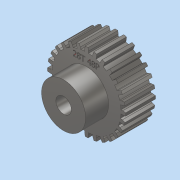
# Autodesk Inventor part: largeIdlerPinion
Saved by Autodesk Inventor 2017 (Build 210142000, 142)
## iProperties
Created: 2016-11-30
Part Number: largeIdlerPinion
Material: Steel, Carbon
Document SubType Name: Modeling
Designer: techn
Density: 7.85 g/cm^3
Appearance: Semi-Polished
Author: techn
Comments: A pinion gear i already own of the 20 to 24 tooth variety - adjust mesh in ballast section based on the axle pitch
Autodesk Inventor part; units mm, degrees
note: some values were not read from the file. Chosen so that the rebuilt part matches the saved one: direction of "Emboss1".
ref_plane "YZ Plane" through (0, 0, 0) normal (1, 0, 0) x (0, 1, 0)
ref_plane "XZ Plane" through (0, 0, 0) normal (0, 1, 0) x (-1, 0, 0)
ref_plane "XY Plane" through (0, 0, 0) normal (0, 0, 1) x (1, 0, 0)
sketch "Sketch1" plane through (0, 0, 0) normal (0, 0, 1) x (1, 0, 0)
  circle A0 centre (0, 0) radius 7.0358
  dimension "d0" = 14.0716
  constraints: 1 centre point, 1 coincident
  measures "d0" diameter of A0
extrude "Extrusion1" add sketch "Sketch1" along normal blind 6.096
sketch "Sketch2" plane through (0, 0, 6.096) normal (0, 0, 1) x (1, 0, 0)
  circle A0 centre (0, 0) radius 4.5085
  dimension "d3" = 9.017
  constraints: 1 centre point, 1 coincident
  measures "d3" diameter of A0
extrude "Extrusion2" add sketch "Sketch2" along normal blind 4.699
sketch "Sketch3" plane through (0, 0, 10.795) normal (0, 0, 1) x (1, 0, 0)
  circle A0 centre (0, 0) radius 1.5875
  dimension "d6" = 3.175
  constraints: 1 centre point, 1 coincident
  measures "d6" diameter of A0
extrude "Extrusion3" cut sketch "Sketch3" against normal blind 25.4
sketch "Sketch5" plane through (0, 0, 0) normal (0, 0, -1) x (-1, 0, 0)
  line L0 (-0.3683, 7.0262) -> (0.3683, 7.0262)
  line L1 (0.3683, 7.0262) -> (0.3683, 7.4072)
  line L2 (0.3683, 7.4072) -> (0.2921, 7.9914)
  line L3 (0.2921, 7.9914) -> (-0.2921, 7.9914)
  line L4 (-0.2921, 7.9914) -> (-0.3683, 7.4072)
  line L5 (-0.3683, 7.4072) -> (-0.3683, 7.0262)
  circle A0 centre (0, 0) radius 7.0358 projected
  point P0 (0, 7.9914)
  point P1 (0, 7.0262)
  dimension "d20" = 0.5842
  dimension "d21" = 0.7366
  dimension "d22" = 0.381
  dimension "d23" = 0.5842
  constraints: 12 end point, 2 midpoint, 2 parallel, 2 vertical alignment, 1 horizontal, 1 horizontal alignment, 1 perpendicular, 2 other
  measures "d20" distance of L2.end L3.end
  measures "d21" distance of L0.start L0.end
  measures "d22" distance of L0.end L1.end
  measures "d23" distance from line of L4.end L3
extrude "Extrusion5" add sketch "Sketch5" against normal up to surface (6.096 mm away) contours A0 L0 | L5 L4 L3 L2 L1 A0 picked at (-0.0409, 7.029)
pattern_circular "Circular Pattern1" count 28 over 360 about axis through (0, 0, 0) along (0, 0, 1) of "Extrusion5"
sketch "Sketch6" plane through (0, 0, 6.096) normal (0, 0, 1) x (1, 0, 0)
  line L0 (-2.8231, 6.1378) -> (2.6097, 6.1378) construction
  line L1 (2.6097, 6.1378) -> (2.6097, 5.0003) construction
  line L2 (2.6097, 5.0003) -> (-2.8231, 5.0003) construction
  line L3 (-2.8231, 5.0003) -> (-2.8231, 6.1378) construction
  line L4 (-2.0727, 5.025) -> (-2.7437, 5.025)
  line L5 (-2.7437, 5.025) -> (-2.7437, 5.1793)
  spline S0 degree 2 poles (-2.7437, 5.1793) (-2.6714, 5.2472) (-2.5427, 5.3733) (-2.4809, 5.4412) knots 0 0 0 1 2 2 2
  spline S1 degree 2 poles (-2.4809, 5.4412) (-2.3566, 5.5779) (-2.2658, 5.7419) (-2.2658, 5.8292) knots 0 0 0 1 2 2 2
  spline S2 degree 2 poles (-2.2658, 5.8292) (-2.2658, 5.875) (-2.294, 5.9438) (-2.3196, 5.9659) knots 0 0 0 1 2 2 2
  spline S3 degree 2 poles (-2.3196, 5.9659) (-2.3451, 5.9879) (-2.4122, 6.01) (-2.4527, 6.01) knots 0 0 0 1 2 2 2
  spline S4 degree 2 poles (-2.4527, 6.01) (-2.4915, 6.01) (-2.5709, 5.9906) (-2.607, 5.9756) knots 0 0 0 1 2 2 2
  spline S5 degree 2 poles (-2.607, 5.9756) (-2.6379, 5.9632) (-2.6952, 5.9279) (-2.7128, 5.9156) knots 0 0 0 1 2 2 2
  line L6 (-2.7128, 5.9156) -> (-2.7208, 5.9156)
  line L7 (-2.7208, 5.9156) -> (-2.7208, 6.0708)
  spline S6 degree 2 poles (-2.7208, 6.0708) (-2.6758, 6.0928) (-2.5144, 6.136) (-2.4421, 6.136) knots 0 0 0 1 2 2 2
  spline S7 degree 2 poles (-2.4421, 6.136) (-2.2896, 6.136) (-2.1176, 5.9747) (-2.1176, 5.8371) knots 0 0 0 1 2 2 2
  spline S8 degree 2 poles (-2.1176, 5.8371) (-2.1176, 5.7727) (-2.1476, 5.6652) (-2.1741, 5.6193) knots 0 0 0 1 2 2 2
  spline S9 degree 2 poles (-2.1741, 5.6193) (-2.2005, 5.5717) (-2.2772, 5.4782) (-2.3196, 5.4333) knots 0 0 0 1 2 2 2
  spline S10 degree 2 poles (-2.3196, 5.4333) (-2.3883, 5.3583) (-2.5568, 5.1978) (-2.607, 5.1511) knots 0 0 0 1 2 2 2
  line L8 (-2.607, 5.1511) -> (-2.0727, 5.1511)
  line L9 (-2.0727, 5.1511) -> (-2.0727, 5.025)
  spline S11 degree 2 poles (-1.5983, 5.0003) (-1.6794, 5.0003) (-1.8125, 5.0488) (-1.8593, 5.0938) knots 0 0 0 1 2 2 2
  spline S12 degree 2 poles (-1.8593, 5.0938) (-1.9051, 5.1379) (-1.9527, 5.2578) (-1.9527, 5.3257) knots 0 0 0 1 2 2 2
  spline S13 degree 2 poles (-1.9527, 5.3257) (-1.9527, 5.4139) (-1.8584, 5.562) (-1.7684, 5.6061) knots 0 0 0 1 2 2 2
  line L10 (-1.7684, 5.6061) -> (-1.7684, 5.6105)
  spline S14 degree 2 poles (-1.7684, 5.6105) (-1.8487, 5.6572) (-1.9263, 5.7683) (-1.9263, 5.8512) knots 0 0 0 1 2 2 2
  spline S15 degree 2 poles (-1.9263, 5.8512) (-1.9263, 5.9738) (-1.7411, 6.1378) (-1.5983, 6.1378) knots 0 0 0 1 2 2 2
  spline S16 degree 2 poles (-1.5983, 6.1378) (-1.4501, 6.1378) (-1.2711, 5.9826) (-1.2711, 5.8609) knots 0 0 0 1 2 2 2
  spline S17 degree 2 poles (-1.2711, 5.8609) (-1.2711, 5.7877) (-1.3566, 5.6449) (-1.4369, 5.6043) knots 0 0 0 1 2 2 2
  line L11 (-1.4369, 5.6043) -> (-1.4369, 5.5999)
  spline S18 degree 2 poles (-1.4369, 5.5999) (-1.3417, 5.5558) (-1.2438, 5.4288) (-1.2438, 5.3283) knots 0 0 0 1 2 2 2
  spline S19 degree 2 poles (-1.2438, 5.3283) (-1.2438, 5.189) (-1.4466, 5.0003) (-1.5983, 5.0003) knots 0 0 0 1 2 2 2
  spline S20 degree 2 poles (-1.3937, 5.3142) (-1.3937, 5.3812) (-1.4466, 5.4606) (-1.5215, 5.5012) knots 0 0 0 1 2 2 2
  spline S21 degree 2 poles (-1.5215, 5.5012) (-1.5462, 5.5153) (-1.6291, 5.5479) (-1.6811, 5.5691) knots 0 0 0 1 2 2 2
  spline S22 degree 2 poles (-1.6811, 5.5691) (-1.7411, 5.5294) (-1.8055, 5.4112) (-1.8055, 5.3363) knots 0 0 0 1 2 2 2
  spline S23 degree 2 poles (-1.8055, 5.3363) (-1.8055, 5.2375) (-1.6864, 5.1088) (-1.5965, 5.1088) knots 0 0 0 1 2 2 2
  spline S24 degree 2 poles (-1.5965, 5.1088) (-1.5048, 5.1088) (-1.3937, 5.219) (-1.3937, 5.3142) knots 0 0 0 1 2 2 2
  spline S25 degree 2 poles (-1.414, 5.8592) (-1.414, 5.9324) (-1.5118, 6.0302) (-1.5991, 6.0302) knots 0 0 0 1 2 2 2
  spline S26 degree 2 poles (-1.5991, 6.0302) (-1.6785, 6.0302) (-1.7799, 5.9429) (-1.7799, 5.868) knots 0 0 0 1 2 2 2
  spline S27 degree 2 poles (-1.7799, 5.868) (-1.7799, 5.8142) (-1.7279, 5.7392) (-1.6759, 5.7093) knots 0 0 0 1 2 2 2
  spline S28 degree 2 poles (-1.6759, 5.7093) (-1.6538, 5.6969) (-1.5603, 5.6537) (-1.5224, 5.6414) knots 0 0 0 1 2 2 2
  spline S29 degree 2 poles (-1.5224, 5.6414) (-1.4589, 5.6899) (-1.414, 5.793) (-1.414, 5.8592) knots 0 0 0 1 2 2 2
  line L12 (-0.8258, 5.025) -> (-0.8258, 5.9844)
  line L13 (-0.8258, 5.9844) -> (-1.1909, 5.9844)
  line L14 (-1.1909, 5.9844) -> (-1.1909, 6.1131)
  line L15 (-1.1909, 6.1131) -> (-0.3161, 6.1131)
  line L16 (-0.3161, 6.1131) -> (-0.3161, 5.9844)
  line L17 (-0.3161, 5.9844) -> (-0.6812, 5.9844)
  line L18 (-0.6812, 5.9844) -> (-0.6812, 5.025)
  line L19 (-0.6812, 5.025) -> (-0.8258, 5.025)
  line L20 (0.9307, 5.3989) -> (0.8011, 5.3989)
  line L21 (0.8011, 5.3989) -> (0.8011, 5.025)
  line L22 (0.8011, 5.025) -> (0.6609, 5.025)
  line L23 (0.6609, 5.025) -> (0.6609, 5.3989)
  line L24 (0.6609, 5.3989) -> (0.1803, 5.3989)
  line L25 (0.1803, 5.3989) -> (0.1803, 5.5523)
  line L26 (0.1803, 5.5523) -> (0.6671, 6.1131)
  line L27 (0.6671, 6.1131) -> (0.8011, 6.1131)
  line L28 (0.8011, 6.1131) -> (0.8011, 5.5161)
  line L29 (0.8011, 5.5161) -> (0.9307, 5.5161)
  line L30 (0.9307, 5.5161) -> (0.9307, 5.3989)
  line L31 (0.6609, 5.5161) -> (0.6609, 5.9412)
  line L32 (0.6609, 5.9412) -> (0.295, 5.5161)
  line L33 (0.295, 5.5161) -> (0.6609, 5.5161)
  spline S30 degree 2 poles (1.376, 5.0003) (1.2949, 5.0003) (1.1618, 5.0488) (1.115, 5.0938) knots 0 0 0 1 2 2 2
  spline S31 degree 2 poles (1.115, 5.0938) (1.0692, 5.1379) (1.0216, 5.2578) (1.0216, 5.3257) knots 0 0 0 1 2 2 2
  spline S32 degree 2 poles (1.0216, 5.3257) (1.0216, 5.4139) (1.1159, 5.562) (1.2059, 5.6061) knots 0 0 0 1 2 2 2
  line L34 (1.2059, 5.6061) -> (1.2059, 5.6105)
  spline S33 degree 2 poles (1.2059, 5.6105) (1.1256, 5.6572) (1.048, 5.7683) (1.048, 5.8512) knots 0 0 0 1 2 2 2
  spline S34 degree 2 poles (1.048, 5.8512) (1.048, 5.9738) (1.2332, 6.1378) (1.376, 6.1378) knots 0 0 0 1 2 2 2
  spline S35 degree 2 poles (1.376, 6.1378) (1.5242, 6.1378) (1.7032, 5.9826) (1.7032, 5.8609) knots 0 0 0 1 2 2 2
  spline S36 degree 2 poles (1.7032, 5.8609) (1.7032, 5.7877) (1.6177, 5.6449) (1.5374, 5.6043) knots 0 0 0 1 2 2 2
  line L35 (1.5374, 5.6043) -> (1.5374, 5.5999)
  spline S37 degree 2 poles (1.5374, 5.5999) (1.6326, 5.5558) (1.7305, 5.4288) (1.7305, 5.3283) knots 0 0 0 1 2 2 2
  spline S38 degree 2 poles (1.7305, 5.3283) (1.7305, 5.189) (1.5277, 5.0003) (1.376, 5.0003) knots 0 0 0 1 2 2 2
  spline S39 degree 2 poles (1.5806, 5.3142) (1.5806, 5.3812) (1.5277, 5.4606) (1.4528, 5.5012) knots 0 0 0 1 2 2 2
  spline S40 degree 2 poles (1.4528, 5.5012) (1.4281, 5.5153) (1.3452, 5.5479) (1.2932, 5.5691) knots 0 0 0 1 2 2 2
  spline S41 degree 2 poles (1.2932, 5.5691) (1.2332, 5.5294) (1.1688, 5.4112) (1.1688, 5.3363) knots 0 0 0 1 2 2 2
  spline S42 degree 2 poles (1.1688, 5.3363) (1.1688, 5.2375) (1.2879, 5.1088) (1.3778, 5.1088) knots 0 0 0 1 2 2 2
  spline S43 degree 2 poles (1.3778, 5.1088) (1.4695, 5.1088) (1.5806, 5.219) (1.5806, 5.3142) knots 0 0 0 1 2 2 2
  spline S44 degree 2 poles (1.5603, 5.8592) (1.5603, 5.9324) (1.4625, 6.0302) (1.3752, 6.0302) knots 0 0 0 1 2 2 2
  spline S45 degree 2 poles (1.3752, 6.0302) (1.2958, 6.0302) (1.1944, 5.9429) (1.1944, 5.868) knots 0 0 0 1 2 2 2
  spline S46 degree 2 poles (1.1944, 5.868) (1.1944, 5.8142) (1.2464, 5.7392) (1.2984, 5.7093) knots 0 0 0 1 2 2 2
  spline S47 degree 2 poles (1.2984, 5.7093) (1.3205, 5.6969) (1.414, 5.6537) (1.4519, 5.6414) knots 0 0 0 1 2 2 2
  spline S48 degree 2 poles (1.4519, 5.6414) (1.5154, 5.6899) (1.5603, 5.793) (1.5603, 5.8592) knots 0 0 0 1 2 2 2
  spline S49 degree 2 poles (2.5823, 5.7851) (2.5823, 5.7146) (2.5321, 5.5876) (2.4871, 5.5435) knots 0 0 0 1 2 2 2
  spline S50 degree 2 poles (2.4871, 5.5435) (2.4307, 5.4879) (2.2781, 5.4306) (2.1617, 5.4306) knots 0 0 0 1 2 2 2
  line L36 (2.1617, 5.4306) -> (2.0391, 5.4306)
  line L37 (2.0391, 5.4306) -> (2.0391, 5.025)
  line L38 (2.0391, 5.025) -> (1.8945, 5.025)
  line L39 (1.8945, 5.025) -> (1.8945, 6.1131)
  line L40 (1.8945, 6.1131) -> (2.1679, 6.1131)
  spline S51 degree 2 poles (2.1679, 6.1131) (2.2649, 6.1131) (2.4007, 6.0814) (2.4527, 6.0452) knots 0 0 0 1 2 2 2
  spline S52 degree 2 poles (2.4527, 6.0452) (2.5136, 6.0038) (2.5823, 5.8759) (2.5823, 5.7851) knots 0 0 0 1 2 2 2
  spline S53 degree 2 poles (2.4315, 5.7807) (2.4315, 5.8371) (2.3928, 5.92) (2.3531, 5.9465) knots 0 0 0 1 2 2 2
  spline S54 degree 2 poles (2.3531, 5.9465) (2.3187, 5.9694) (2.227, 5.9879) (2.1591, 5.9879) knots 0 0 0 1 2 2 2
  line L41 (2.1591, 5.9879) -> (2.0391, 5.9879)
  line L42 (2.0391, 5.9879) -> (2.0391, 5.5541)
  line L43 (2.0391, 5.5541) -> (2.1379, 5.5541)
  spline S55 degree 2 poles (2.1379, 5.5541) (2.2261, 5.5541) (2.3346, 5.5823) (2.3698, 5.6193) knots 0 0 0 1 2 2 2
  spline S56 degree 2 poles (2.3698, 5.6193) (2.4024, 5.6519) (2.4315, 5.7287) (2.4315, 5.7807) knots 0 0 0 1 2 2 2
  point P0 (0, 0)
  constraints: 2 other
emboss "Emboss1" sketch "Sketch6" operation cut depth 0.254 direction (0, 0, -1)
body "Solid1"
